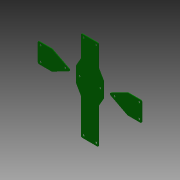
# Autodesk Inventor part: Bottom Plate Veroboard
Saved by Autodesk Inventor 2015 (Build 190159000, 159)
## iProperties
Created: 2015-11-27
Part Number: Bottom Plate Veroboard
Material: ABS Plastic
Document SubType Name: Modeling
Designer: James
Density: 1.06 g/cm^3
Appearance: Smooth - White
Author: James
Autodesk Inventor part; units mm, degrees
ref_plane "YZ Plane" through (0, 0, 0) normal (1, 0, 0) x (0, 1, 0)
ref_plane "XZ Plane" through (0, 0, 0) normal (0, 1, 0) x (-1, 0, 0)
ref_plane "XY Plane" through (0, 0, 0) normal (0, 0, 1) x (1, 0, 0)
sketch "Sketch1" plane through (0, 0, 0) normal (0, 1, 0) x (-1, 0, 0)
  line L0 (-49.1414, 1.7802) -> (-66.9436, 10.8951)
  line L1 (-66.9436, -10.8951) -> (-49.1414, -1.7802)
  line L2 (-37.6128, -11.7654) -> (-37.6128, 11.7654)
  line L3 (5, 11.7654) -> (5, -11.7654)
  line L4 (4.7321, -12.7654) -> (-2.2321, -24.8275)
  line L5 (-37.3449, -12.7654) -> (-30.3808, -24.8275)
  line L6 (-37.3449, 12.7654) -> (-30.3808, 24.8275)
  line L7 (4.7321, 12.7654) -> (-2.2321, 24.8275)
  line L8 (-2.5, 25.8275) -> (-2.5, 57.6025)
  line L9 (-30.1128, 25.8275) -> (-30.1128, 57.6025)
  line L10 (-28.1128, -81.6025) -> (-4.5, -81.6025)
  line L11 (-30.1128, -25.8275) -> (-30.1128, -79.6025)
  line L12 (-2.5, -79.6025) -> (-2.5, -25.8275)
  line L13 (-28.1128, 59.6025) -> (-4.5, 59.6025)
  arc A0 (-28.1128, 59.6025) -> (-30.1128, 57.6025) centre (-28.1128, 57.6025) ccw
  arc A1 (-2.5, 57.6025) -> (-4.5, 59.6025) centre (-4.5, 57.6025) ccw
  arc A2 (-2.5, 25.8275) -> (-2.2321, 24.8275) centre (-0.5, 25.8275) ccw
  arc A3 (5, 11.7654) -> (4.7321, 12.7654) centre (3, 11.7654) ccw
  arc A4 (4.7321, -12.7654) -> (5, -11.7654) centre (3, -11.7654) ccw
  arc A5 (-2.2321, -24.8275) -> (-2.5, -25.8275) centre (-0.5, -25.8275) ccw
  arc A6 (-30.1128, -25.8275) -> (-30.3808, -24.8275) centre (-32.1128, -25.8275) ccw
  arc A7 (-37.6128, -11.7654) -> (-37.3449, -12.7654) centre (-35.6128, -11.7654) ccw
  arc A8 (-37.3449, 12.7654) -> (-37.6128, 11.7654) centre (-35.6128, 11.7654) ccw
  arc A9 (-30.3808, 24.8275) -> (-30.1128, 25.8275) centre (-32.1128, 25.8275) ccw
  arc A10 (-4.5, -81.6025) -> (-2.5, -79.6025) centre (-4.5, -79.6025) ccw
  arc A11 (-30.1128, -79.6025) -> (-28.1128, -81.6025) centre (-28.1128, -79.6025) ccw
  arc A12 (-49.1414, -1.7802) -> (-49.1414, 1.7802) centre (-50.0529, 0) ccw
  line L14 (-66.9436, 10.8951) -> (-75.4155, 15.2328)
  line L15 (-76.327, 15.4526) -> (-95.8447, 15.4526)
  line L16 (-66.9436, -10.8951) -> (-75.4155, -15.2328)
  line L17 (-76.327, -15.4526) -> (-95.8447, -15.4526)
  line L18 (-97.8447, -13.4526) -> (-97.8447, 13.4526)
  arc A13 (-95.8447, 15.4526) -> (-97.8447, 13.4526) centre (-95.8447, 13.4526) ccw
  arc A14 (-75.4155, 15.2328) -> (-76.327, 15.4526) centre (-76.327, 13.4526) ccw
  arc A15 (-76.327, -15.4526) -> (-75.4155, -15.2328) centre (-76.327, -13.4526) ccw
  arc A16 (-97.8447, -13.4526) -> (-95.8447, -15.4526) centre (-95.8447, -13.4526) ccw
  line L19 (16.5286, 1.7802) -> (34.3308, 10.8951)
  arc A17 (16.5286, 1.7802) -> (16.5286, -1.7802) centre (17.4401, 0) ccw
  line L20 (34.3308, -10.8951) -> (16.5286, -1.7802)
  line L21 (34.3308, 10.8951) -> (42.8026, 15.2328)
  arc A18 (43.7141, 15.4526) -> (42.8026, 15.2328) centre (43.7141, 13.4526) ccw
  line L22 (43.7141, 15.4526) -> (63.2319, 15.4526)
  line L23 (34.3308, -10.8951) -> (42.8026, -15.2328)
  line L24 (43.7141, -15.4526) -> (63.2319, -15.4526)
  arc A19 (42.8026, -15.2328) -> (43.7141, -15.4526) centre (43.7141, -13.4526) ccw
  line L25 (65.2319, -13.4526) -> (65.2319, 13.4526)
  arc A20 (63.2319, -15.4526) -> (65.2319, -13.4526) centre (63.2319, -13.4526) ccw
  arc A21 (65.2319, 13.4526) -> (63.2319, 15.4526) centre (63.2319, 13.4526) ccw
  circle A22 centre (-26.1128, -77.6025) radius 1.6
  circle A23 centre (-6.5, -77.6025) radius 1.6
  circle A24 centre (-32.6128, 0) radius 1.6
  circle A25 centre (0, 0) radius 1.6
  circle A26 centre (-26.1128, 55.6025) radius 1.6
  circle A27 centre (-6.5, 55.6025) radius 1.6
  circle A28 centre (-93.8447, 11.4526) radius 1.6
  circle A29 centre (-93.8447, -11.4526) radius 1.6
  circle A30 centre (-55.0529, 0) radius 1.6
  circle A31 centre (61.2319, 11.4526) radius 1.6
  circle A32 centre (61.2319, -11.4526) radius 1.6
  circle A33 centre (22.4401, 0) radius 1.6
  constraints: 52 end point, 44 point on circle, 34 centre point
extrude "Extrusion1" add sketch "Sketch1" along normal blind 1
body "Solid1"
